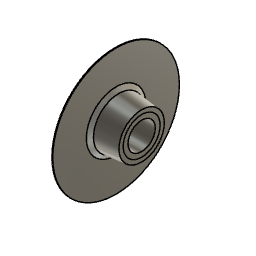
RIN_1 (Autodesk Fusion 360 design; units mm, degrees)
Autodesk Fusion 360 part; units mm, degrees
sketch "Boceto1" plane through (0, 0, 0) normal (0, 0, 1) x (1, 0, 0)
  line L0 (0, 44) -> (-55.2981, 57.8245)
  line L1 (-55.2981, 57.8245) -> (-62.9274, 70.7394)
  line L2 (-60.9274, 70.7394) -> (-54.6242, 60.0694)
  line L3 (-54.6242, 60.0694) -> (0, 54)
  line L4 (0, 54) -> (0, 44)
  line L5 (-62.9274, 70.7394) -> (-62.9274, 150.7394)
  line L6 (-62.9274, 150.7394) -> (-60.9274, 150.7394)
  line L7 (-60.9274, 150.7394) -> (-60.9274, 70.7394)
  dimension "d37" = 57
  dimension "d38" = 15
  dimension "d40" = 54.6242
  dimension "d43" = 80
  dimension "d44" = 2
  constraint parallel L1 L2
  constraint vertical L4
  constraint vertical L5
  constraint perpendicular L5 L6
  constraint perpendicular L6 L7
  measures "d37" distance of L0.start L0.end
  measures "d38" distance of L0.end L1.end
  measures "d40" horizontal distance of L2.end L3.end
  measures "d43" distance of L1.end L5.end
  measures "d44" distance of L5.end L6.end
revolve "Revolución1" add sketch "Boceto1" angle 360 about axis through (1.75, 0, 0) along (1, 0, 0) makes body 1
sketch "Boceto5" plane through (0, 0, 0) normal (1, 0, 0) x (0, 1, 0)
  circle A0 centre (0, 0) radius 44
  dimension "d46" = 88
  constraint coincident A0.centre origin
  measures "d46" diameter of A0
extrude "Extruir1" add sketch "Boceto5" against normal blind 15 separate body makes body 2
extrude "Extruir2" add 1 faces at (-15, 11.6304, -6.1249) along direction (-1, 0, 0) blind 50 on bodies 2 bodies 2
combine "Combinar1" operation add target body 2 tool bodies 1
sketch "Boceto6" plane through (0, 0, 0) normal (1, 0, 0) x (0, 1, 0)
  circle A0 centre (0, 0) radius 32.5
  dimension "d51" = 65
  constraint coincident A0.centre origin
  measures "d51" diameter of A0
extrude "Extruir3" cut sketch "Boceto6" against normal blind 50 bodies 2
sketch "Boceto7" plane through (-50, 0, 0) normal (1, 0, 0) x (0, 1, 0)
  circle A0 centre (0, 0) radius 32.5
  circle A1 centre (0, 0) radius 4.25
  dimension "d54" = 8.5
  constraint coincident A0.centre A1.centre
  measures "d54" diameter of A1
extrude "Extruir4" cut sketch "Boceto7" against normal blind 15 contours A1 bodies 2
named bodies: "Cuerpo1"
